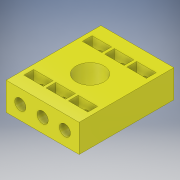
# Autodesk Inventor part: 000.406 - Проставка
Saved by Autodesk Inventor 2019 (Build 230136000, 136)
## iProperties
Created: 2020-02-29
Part Number: 000.406 - Проставка
Material: Пластик АБС
Document SubType Name: Modeling
Designer: Петров Иван
Density: 1.06 g/cm^3
Appearance: Желтый
Author: Петров Иван
Autodesk Inventor part; units mm, degrees
ref_plane "YZ Plane" through (0, 0, 0) normal (1, 0, 0) x (0, 1, 0)
ref_plane "XZ Plane" through (0, 0, 0) normal (0, 1, 0) x (-1, 0, 0)
ref_plane "XY Plane" through (0, 0, 0) normal (0, 0, 1) x (1, 0, 0)
sketch "Эскиз1" plane through (0, 0, 0) normal (0, 1, 0) x (-1, 0, 0)
  line L0 (-13.1, 17) -> (13.1, 17)
  line L1 (13.1, 17) -> (13.1, -17)
  line L2 (13.1, -17) -> (-13.1, -17)
  line L3 (-13.1, -17) -> (-13.1, 17)
  line L4 (-13.1, 17) -> (13.1, -17) construction
  line L5 (13.1, 17) -> (-13.1, -17) construction
  point P0 (0, 0)
  dimension "d0" = 26.2
  dimension "d1" = 34
  constraints: 12 end point, 2 midpoint, 2 parallel, 1 horizontal, 1 perpendicular
  measures "d0" distance of L1.end L2.end
  measures "d1" distance of L0.end L1.end
extrude "Выдавливание1" add sketch "Эскиз1" along normal blind 10
sketch "Эскиз2" plane through (-13.1, 0, 17) normal (0, 0, 1) x (1, 0, 0)
  line L0 (0, 10) -> (26.2, 10) projected
  line L1 (13.1, 10) -> (13.1, 5)
  circle A0 centre (13.1, 5) radius 2
  point P0 (13.1, 0)
  dimension "d4" = 5
  dimension "d5" = 4
  constraints: 2 end point, 1 centre point, 1 coincident, 1 midpoint, 1 vertical
  measures "d4" distance of L1.start L1.end
  measures "d5" diameter of A0
extrude "Выдавливание2" cut sketch "Эскиз2" against normal blind 10
sketch "Эскиз4" plane through (0, 10, 0) normal (0, 1, 0) x (1, 0, 0)
  line L0 (2, -7) -> (-2, -7) projected
  line L1 (3.4971, -12.25) -> (-3.4971, -12.25)
  line L2 (-3.4971, -12.25) -> (-3.4971, -8.75)
  line L3 (-3.4971, -8.75) -> (3.4971, -8.75)
  line L4 (3.4971, -8.75) -> (3.4971, -12.25)
  line L5 (3.4971, -12.25) -> (-3.4971, -8.75) construction
  line L6 (-3.4971, -12.25) -> (3.4971, -8.75) construction
  point P0 (0, 0)
  point P1 (0, -10.5)
  dimension "d20" = 10.5
  constraints: 12 end point, 2 midpoint, 2 parallel, 1 perpendicular
  measures "d20" distance of point (0, 0) point (0, -10.5)
extrude "Выдавливание3" cut sketch "Эскиз4" against normal through all
pattern_linear "Прямоуг.массив2" count 3 spacing 8 along (1, 0, 0) of "Выдавливание2", "Выдавливание3" first direction both ways yes
mirror "Зеркальное отражение2" about plane through (0, 0, 0) normal (0, 0, 1) of "Выдавливание2", "Выдавливание3", "Прямоуг.массив2"
sketch "Эскиз5" plane through (0, 10, 0) normal (0, 1, 0) x (1, 0, 0)
  circle A0 centre (0, 0) radius 5
  dimension "d17" = 10
  constraints: 1 centre point, 1 coincident
  measures "d17" diameter of A0
extrude "Выдавливание4" cut sketch "Эскиз5" against normal blind 10
sketch "Эскиз6" plane through (0, 10, 0) normal (0, 1, 0) x (1, 0, 0)
  circle A0 centre (0, 0) radius 5 projected
  line L0 (4.5029, 8.75) -> (4.5029, 12.25) projected
  line L1 (4.5029, 12.25) -> (11.4971, 12.25) projected
  line L2 (11.4971, 12.25) -> (11.4971, 8.75) projected
  line L3 (-11.4971, 8.75) -> (-11.4971, 12.25) projected
  line L4 (-11.4971, 12.25) -> (-4.5029, 12.25) projected
  line L5 (-4.5029, 12.25) -> (-4.5029, 8.75) projected
  line L6 (-3.4971, 8.75) -> (-3.4971, 12.25) projected
  line L7 (-3.4971, 12.25) -> (3.4971, 12.25) projected
  line L8 (3.4971, 12.25) -> (3.4971, 8.75) projected
  line L9 (4.5029, -12.25) -> (4.5029, -8.75) projected
  line L10 (11.4971, -8.75) -> (11.4971, -12.25) projected
  line L11 (11.4971, -12.25) -> (4.5029, -12.25) projected
  line L12 (-11.4971, -12.25) -> (-11.4971, -8.75) projected
  line L13 (-4.5029, -8.75) -> (-4.5029, -12.25) projected
  line L14 (-4.5029, -12.25) -> (-11.4971, -12.25) projected
  line L15 (3.4971, -8.75) -> (3.4971, -12.25) projected
  line L16 (3.4971, -12.25) -> (-3.4971, -12.25) projected
  line L17 (-3.4971, -12.25) -> (-3.4971, -8.75) projected
  line L18 (-13.1, -17) -> (13.1, -17) projected
  line L19 (13.1, -17) -> (13.1, 17) projected
  line L20 (13.1, 17) -> (-13.1, 17) projected
  line L21 (-13.1, 17) -> (-13.1, -17) projected
  line L22 (11.4971, 8.75) -> (4.5029, 8.75) projected
  line L23 (-4.5029, 8.75) -> (-11.4971, 8.75) projected
  line L24 (3.4971, 8.75) -> (-3.4971, 8.75) projected
  line L25 (4.5029, -8.75) -> (11.4971, -8.75) projected
  line L26 (-11.4971, -8.75) -> (-4.5029, -8.75) projected
  line L27 (-3.4971, -8.75) -> (3.4971, -8.75) projected
